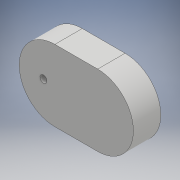
# Autodesk Inventor part: 071_0202_RollCutter20mmCenter
Saved by Autodesk Inventor 2018 (Build 220112000, 112)
## iProperties
Created: 2018-07-06
Part Number: 071_0202_RollCutter20mmCenter
Material: Generic
Document SubType Name: Modeling
Designer: deniz
Density: 1 g/cm^3
Appearance: Default
Author: deniz
Autodesk Inventor part; units mm, degrees
ref_plane "YZ Plane" through (0, 0, 0) normal (1, 0, 0) x (0, 1, 0)
ref_plane "XZ Plane" through (0, 0, 0) normal (0, 1, 0) x (-1, 0, 0)
ref_plane "XY Plane" through (0, 0, 0) normal (0, 0, 1) x (1, 0, 0)
sketch "Sketch1" plane through (0, 0, 0) normal (0, 1, 0) x (-1, 0, 0)
  line L0 (0, 0) -> (-30, 0) construction
  line L1 (0, 25) -> (-30, 25)
  line L2 (-30, -25) -> (0, -25)
  arc A0 (0, -25) -> (0, 25) centre (0, 0) ccw
  arc A1 (-30, 25) -> (-30, -25) centre (-30, 0) ccw
  circle A2 centre (8, 0) radius 2.45
  line L3 (0, 0) -> (25, 0) construction
  circle A3 centre (8, 0) radius 22.5 construction
  circle A4 centre (8, 0) radius 15 construction
  point P0 (-15, 0)
  dimension "d26" = 50
  dimension "d27" = 30
  dimension "d28" = 4.9
  dimension "d29" = 8
  dimension "d30" = 17
  dimension "d31" = 45
  dimension "d32" = 30
  constraints: 10 end point, 5 centre point, 5 point on circle, 4 tangent, 3 coincident, 1 horizontal, 1 midpoint, 1 parallel, 1 point on line
  measures "d26" diameter of A0
  measures "d27" distance of L0.start L0.end
  measures "d28" diameter of A2
  measures "d29" distance of A2.centre point (0, 0)
  measures "d30" distance of L3.end A2.centre
  measures "d31" diameter of A3
  measures "d32" diameter of A4
extrude "Extrusion6" add sketch "Sketch1" along normal blind 19.2
equation "\"d23\" = printing_w"
equation "\"blade_w\" = 0.3"
equation "\"calib_w\" = 0.3"
equation "\"print_fit_w\" = 0.2"
equation "\"printing_w\" = -calib_w + nominal_w - blade_w - print_fit_w"
equation "\"nominal_w\" = 20"
body "Solid3"
